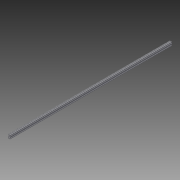
# Autodesk Inventor part: makerslide_1800
Saved by Autodesk Inventor 2013 (Build 170138000, 138)
## iProperties
Created: 2013-06-20
Part Number: makerslide_1800
Material: Generic
Document SubType Name: Modeling
Designer: Brett
Density: 1 g/cm^3
Author: Brett
Autodesk Inventor part; units mm, degrees
ref_plane "YZ Plane" through (0, 0, 0) normal (1, 0, 0) x (0, 1, 0)
ref_plane "XZ Plane" through (0, 0, 0) normal (0, 1, 0) x (-1, 0, 0)
ref_plane "XY Plane" through (0, 0, 0) normal (0, 0, 1) x (1, 0, 0)
sketch "Sketch1" plane through (0, 0, 0) normal (0, 0, 1) x (1, 0, 0)
  arc A0 (-12.375, -10.5929) -> (-12.2286, -10.9464) centre (-11.875, -10.5929) ccw
  line L0 (-12.2286, -10.9464) -> (-10.3536, -12.8214)
  arc A1 (-10.3536, -12.8214) -> (-9.6464, -12.8214) centre (-10, -12.4679) ccw
  line L1 (-9.6464, -12.8214) -> (-7.7714, -10.9464)
  arc A2 (-7.7714, -10.9464) -> (-7.625, -10.5929) centre (-8.125, -10.5929) ccw
  line L2 (-7.625, -10.5929) -> (-7.625, -10.5)
  arc A3 (-7.125, -10) -> (-7.625, -10.5) centre (-7.125, -10.5) ccw
  line L3 (-7.125, -10) -> (-3.3, -10)
  arc A4 (-3.3, -10) -> (-3, -9.7) centre (-3.3, -9.7) ccw
  line L4 (-3, -9.7) -> (-3, -8)
  line L5 (-3, -8) -> (-6, -8)
  line L6 (-6, -8) -> (-6, -7.0607)
  line L7 (-6, -7.0607) -> (-2.9393, -4)
  line L8 (-2.9393, -4) -> (-0.3, -4)
  line L9 (-0.3, -4) -> (0, -3.7)
  line L10 (0, -3.7) -> (0.3, -4)
  line L11 (0.3, -4) -> (2.9393, -4)
  line L12 (2.9393, -4) -> (6, -7.0607)
  line L13 (6, -7.0607) -> (6, -8)
  line L14 (6, -8) -> (3, -8)
  line L15 (3, -8) -> (3, -9.7)
  arc A5 (3, -9.7) -> (3.3, -10) centre (3.3, -9.7) ccw
  line L16 (3.3, -10) -> (9, -10)
  arc A6 (9, -10) -> (10, -9) centre (9, -9) ccw
  line L17 (10, -9) -> (10, -3.3)
  arc A7 (10, -3.3) -> (9.7, -3) centre (9.7, -3.3) ccw
  line L18 (9.7, -3) -> (8, -3)
  line L19 (8, -3) -> (8, -6)
  line L20 (8, -6) -> (7.0607, -6)
  line L21 (7.0607, -6) -> (4, -2.9393)
  line L22 (4, -2.9393) -> (4, -0.3)
  line L23 (4, -0.3) -> (3.7, 0)
  line L24 (3.7, 0) -> (4, 0.3)
  line L25 (4, 0.3) -> (4, 2.9393)
  line L26 (4, 2.9393) -> (7.0607, 6)
  line L27 (7.0607, 6) -> (8, 6)
  line L28 (8, 6) -> (8, 3)
  line L29 (8, 3) -> (9.7, 3)
  arc A8 (9.7, 3) -> (10, 3.3) centre (9.7, 3.3) ccw
  line L30 (10, 3.3) -> (10, 16.7)
  arc A9 (10, 16.7) -> (9.7, 17) centre (9.7, 16.7) ccw
  line L31 (9.7, 17) -> (8, 17)
  line L32 (8, 17) -> (8, 14)
  line L33 (8, 14) -> (7.0607, 14)
  line L34 (7.0607, 14) -> (4, 17.0607)
  line L35 (4, 17.0607) -> (4, 19.7)
  line L36 (4, 19.7) -> (3.7, 20)
  line L37 (3.7, 20) -> (4, 20.3)
  line L38 (4, 20.3) -> (4, 22.9393)
  line L39 (4, 22.9393) -> (7.0607, 26)
  line L40 (7.0607, 26) -> (8, 26)
  line L41 (8, 26) -> (8, 23)
  line L42 (8, 23) -> (9.7, 23)
  arc A10 (9.7, 23) -> (10, 23.3) centre (9.7, 23.3) ccw
  line L43 (10, 23.3) -> (10, 29)
  arc A11 (10, 29) -> (9, 30) centre (9, 29) ccw
  line L44 (9, 30) -> (3.3, 30)
  arc A12 (3.3, 30) -> (3, 29.7) centre (3.3, 29.7) ccw
  line L45 (3, 29.7) -> (3, 28)
  line L46 (3, 28) -> (6, 28)
  line L47 (6, 28) -> (6, 27.0607)
  line L48 (6, 27.0607) -> (2.9393, 24)
  line L49 (2.9393, 24) -> (0.3, 24)
  line L50 (0.3, 24) -> (0, 23.7)
  line L51 (0, 23.7) -> (-0.3, 24)
  line L52 (-0.3, 24) -> (-2.9393, 24)
  line L53 (-2.9393, 24) -> (-6, 27.0607)
  line L54 (-6, 27.0607) -> (-6, 28)
  line L55 (-6, 28) -> (-3, 28)
  line L56 (-3, 28) -> (-3, 29.7)
  arc A13 (-3, 29.7) -> (-3.3, 30) centre (-3.3, 29.7) ccw
  line L57 (-3.3, 30) -> (-7.125, 30)
  arc A14 (-7.625, 30.5) -> (-7.125, 30) centre (-7.125, 30.5) ccw
  line L58 (-7.625, 30.5) -> (-7.625, 30.5929)
  arc A15 (-7.625, 30.5929) -> (-7.7714, 30.9464) centre (-8.125, 30.5929) ccw
  line L59 (-7.7714, 30.9464) -> (-9.6464, 32.8214)
  arc A16 (-9.6464, 32.8214) -> (-10.3536, 32.8214) centre (-10, 32.4679) ccw
  line L60 (-10.3536, 32.8214) -> (-12.2286, 30.9464)
  arc A17 (-12.2286, 30.9464) -> (-12.375, 30.5929) centre (-11.875, 30.5929) ccw
  line L61 (-12.375, 30.5929) -> (-12.375, 30)
  line L62 (-12.375, 30) -> (-10, 30)
  line L63 (-10, 30) -> (-10, 23.3)
  arc A18 (-10, 23.3) -> (-9.7, 23) centre (-9.7, 23.3) ccw
  line L64 (-9.7, 23) -> (-8, 23)
  line L65 (-8, 23) -> (-8, 26)
  line L66 (-8, 26) -> (-7.0607, 26)
  line L67 (-7.0607, 26) -> (-4, 22.9393)
  line L68 (-4, 22.9393) -> (-4, 20.3)
  line L69 (-4, 20.3) -> (-3.7, 20)
  line L70 (-3.7, 20) -> (-4, 19.7)
  line L71 (-4, 19.7) -> (-4, 17.0607)
  line L72 (-4, 17.0607) -> (-7.0607, 14)
  line L73 (-7.0607, 14) -> (-8, 14)
  line L74 (-8, 14) -> (-8, 17)
  line L75 (-8, 17) -> (-9.7, 17)
  arc A19 (-9.7, 17) -> (-10, 16.7) centre (-9.7, 16.7) ccw
  line L76 (-10, 16.7) -> (-10, 0.3)
  line L77 (-10, 0.3) -> (-9.7, 0)
  line L78 (-9.7, 0) -> (-10, -0.3)
  line L79 (-10, -0.3) -> (-10, -10)
  line L80 (-10, -10) -> (-12.375, -10)
  line L81 (-12.375, -10) -> (-12.375, -10.5929)
  line L82 (6.4393, 12.5) -> (8, 12.5)
  line L83 (8, 12.5) -> (8, 7.5)
  line L84 (8, 7.5) -> (6.4393, 7.5)
  line L85 (6.4393, 7.5) -> (2.9393, 4)
  line L86 (2.9393, 4) -> (-2.9393, 4)
  line L87 (-2.9393, 4) -> (-6.4393, 7.5)
  line L88 (-6.4393, 7.5) -> (-8, 7.5)
  line L89 (-8, 7.5) -> (-8, 12.5)
  line L90 (-8, 12.5) -> (-6.4393, 12.5)
  line L91 (-6.4393, 12.5) -> (-2.9393, 16)
  line L92 (-2.9393, 16) -> (2.9393, 16)
  line L93 (2.9393, 16) -> (6.4393, 12.5)
  line L94 (-7.0607, -6) -> (-8, -6)
  line L95 (-8, -6) -> (-8, 6)
  line L96 (-8, 6) -> (-7.0607, 6)
  line L97 (-7.0607, 6) -> (-4, 2.9393)
  line L98 (-4, 2.9393) -> (-4, -2.9393)
  line L99 (-4, -2.9393) -> (-7.0607, -6)
  circle A20 centre (0, 20) radius 2.1
  circle A21 centre (0, 0) radius 2.1
  constraints: 200 end point, 76 tangent, 51 parallel, 40 point on circle, 28 perpendicular, 22 centre point, 18 equal radius, 6 collinear
extrude "Extrusion1" add sketch "Sketch1" along normal blind 1800
body "Solid1"
